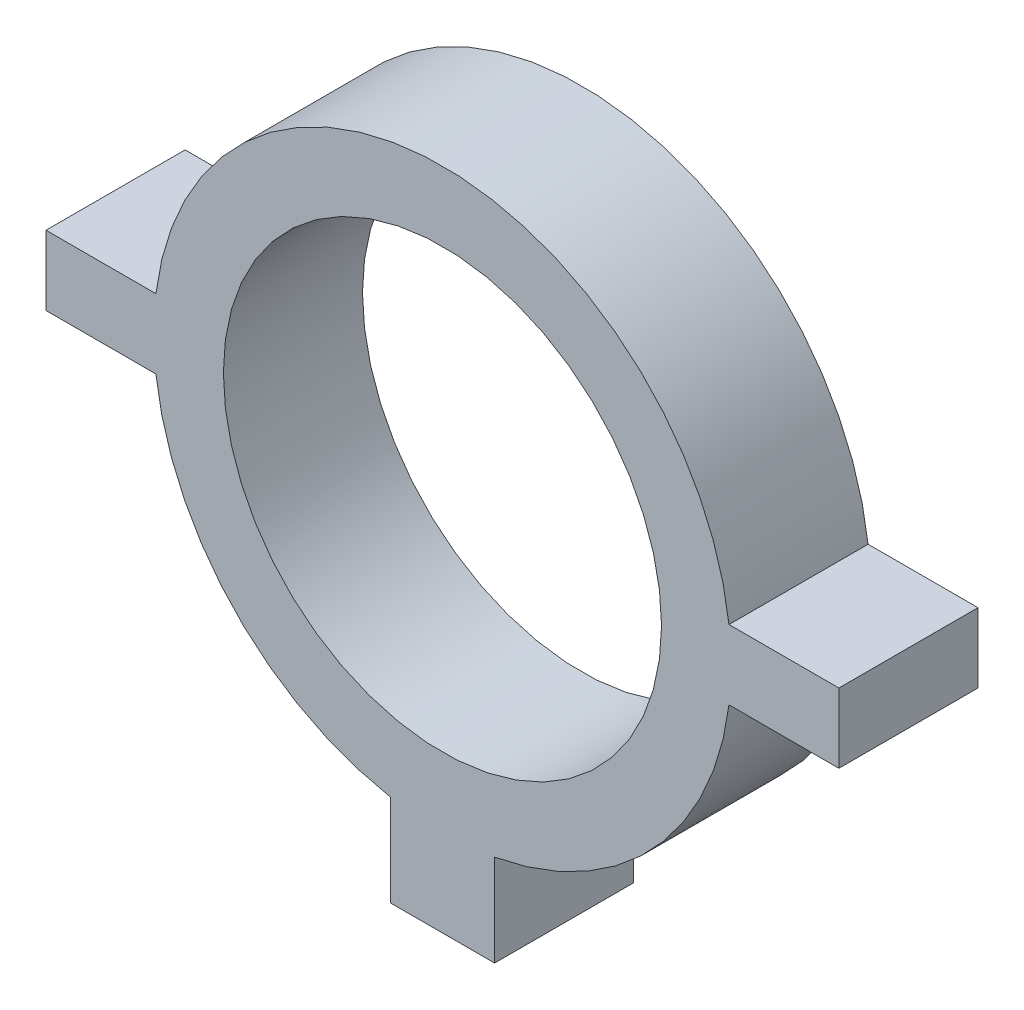
# Autodesk Inventor part: Pipe clamp bracket
Saved by Autodesk Inventor 2025.4 (Build 294407000, 407)
## iProperties
Created: 2026-02-10
Part Number: Pipe clamp bracket
Material: Generic
Document SubType Name: Modeling
Designer: admin
Density: 1 g/cm^3
Appearance: Default
Author: admin
Autodesk Inventor part; units mm, degrees
ref_plane "YZ Plane" through (0, 0, 0) normal (1, 0, 0) x (0, 1, 0)
ref_plane "XZ Plane" through (0, 0, 0) normal (0, 1, 0) x (-1, 0, 0)
ref_plane "XY Plane" through (0, 0, 0) normal (0, 0, 1) x (1, 0, 0)
sketch "Sketch1" plane through (0, 0, 0) normal (0, 0, 1) x (1, 0, 0)
  circle A0 centre (0, 54) radius 31.5
  circle A1 centre (0, 54) radius 41.5
  line L0 (57, 49) -> (-57, 49)
  line L1 (-57, 49) -> (-57, 59)
  line L2 (-57, 59) -> (57, 59)
  line L3 (57, 59) -> (57, 49)
  line L4 (57, 49) -> (-57, 59) construction
  line L5 (-57, 49) -> (57, 59) construction
  line L6 (-7.5, 0) -> (7.5, 0)
  line L7 (7.5, 0) -> (7.5, 22.5)
  line L8 (7.5, 22.5) -> (-7.5, 22.5) construction
  line L9 (-7.5, 22.5) -> (-7.5, 0)
  point P0 (0, 0)
  point P1 (0, 0)
  point P2 (41.1977, 49)
  point P3 (41.1977, 59)
  point P4 (-41.1977, 59)
  point P5 (-41.1977, 49)
  point P6 (-7.5, 13.1833)
  point P7 (7.5, 13.1833)
  dimension "d0" = 54
  dimension "d2" = 10
  dimension "d3" = 63
  dimension "d4" = 10
  dimension "d5" = 114
  dimension "d6" = 15
  constraints: 20 end point, 4 parallel, 3 midpoint, 2 centre point, 2 coincident, 2 horizontal, 2 perpendicular, 1 tangent, 1 vertical alignment
  measures "d0" distance of point (0, 0) A0.centre
  measures "d2" radial gap between concentric circles of A1 A0
  measures "d3" diameter of A0
  measures "d4" distance of L2.end L0.start
  measures "d5" distance of L1.end L2.end
  measures "d6" distance between parallel lines of L7 L9
extrude "Extrusion1" add sketch "Sketch1" along normal mid plane 20 contours A0 L2 A1 L0 | A0 L2 A1 | L0 A1 A0 | A0 L0 A1 L2 | L2 L3 L0 A1 | A1 L0 L1 L2 | L7 L6 L9 A1
equation "\"d4\" = d2"
body "Solid1"
